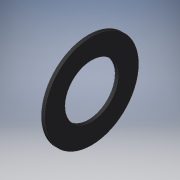
# Autodesk Inventor part: washer_BA1730
Saved by Autodesk Inventor 2019 (Build 230136000, 136)
## iProperties
Created: 2023-09-05
Part Number: washer_BA1730
Material: Generic
Catalog Web Link: www.cadenas.de
Description: BA_ _ _ _ __washer-Thrust Needle Roller Bearings with Retainers
Vendor: MISUMI
Document SubType Name: Modeling
Designer: psAdmin
Manufacturer: MISUMI
Mass: 0.479878 g
Surface Area: 11.0741 cm^2
Volume: 0.479878 cm^3
Density: 1 g/cm^3
Appearance: PSOLRGB-175-175-175
Category: PARTsolutions
Company: MISUMI
Title: washer_BA1730
Author: Cadenas PARTsolutions
Comments: Thrust Needle Roller Bearings with Retainers
PSOL_IDENT_0: {$CADENAS_DATA/23d-libs/misumi/metric/12_bearing_holders/washer_ba1024.prj},178 {VTYP=3D},{NB=washer
PSOL_IDENT_1: _BA1730},{LINA=washer_BA1730},{NN=BA_ _ _ _ __washer},{DATE=19.10.2020 20:02:28},{GEOMDATE=19.10.202
PSOL_IDENT_2: 0 19:34:46},{VERSION=},{LINEID=40},{WBVAR=},{WBNUMERIC=}  {NB=washer_BA1730},{LINA=washer_BA1730},{K
PSOL_IDENT_3: T=DUMMY},{TYPE=BA1730},{DD=17},{D=30},{B=2},{F=29.0},{F1=19.0},{DD1=17},{D1=30},{B1=1}
NB: washer_BA1730
NN: BA_ _ _ _ __washer
NT: Thrust Needle Roller Bearings with Retainers
NBSYN: washer_$TYPE.
LINA: washer_BA1730
CATALOG: Misumi
TYPE: BA1730
DD: 17
D: 30
B: 2
F: 29
F1: 19
DD1: 17
D1: 30
B1: 1
SUPPLIER: MISUMI
ARTICLENO: washer_BA1730
BOMINFO: washer_BA1730
CREATOR: CADENAS GmbH
Autodesk Inventor part; units mm, degrees
sketch "Sketch_1" plane through (0, 0, 0) normal (0, 0, 1) x (1, 0, 0)
  line L0 (50, 0) -> (-50, 0)
  line L1 (-0.5, 15) -> (-0.5, 8.5)
  line L2 (-0.5, 8.5) -> (0.5, 8.5)
  line L3 (0.5, 8.5) -> (0.5, 15)
  line L4 (0.5, 15) -> (-0.5, 15)
  constraints: 10 end point
revolve "Revolution1" add sketch "Sketch_1" angle 360 about axis through (50, 0, 0) along (1, 0, 0)
ref_plane "washer1_XY" through (0, 0, 0) normal (1, 0, 0) x (0, 0, -1)
ref_plane "washer1_YZ" through (0, 0, 0) normal (0, 0, -1) x (0, 1, 0)
ref_plane "washer1_ZX" through (0, 0, 0) normal (0, 1, 0) x (1, 0, 0)
ref_plane "washer2_XY" through (0, 0, 0) normal (1, 0, 0) x (0, 0, -1)
ref_plane "washer2_YZ" through (0, 0, 0) normal (0, 0, -1) x (0, 1, 0)
ref_plane "washer2_ZX" through (0, 0, 0) normal (0, 1, 0) x (1, 0, 0)
body "Solid1"
